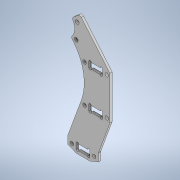
# Autodesk Inventor part: 頭_メインフレーム
Saved by Autodesk Inventor 2020 (Build 240168000, 168)
## iProperties
Created: 2021-09-02
Part Number: 頭_メインフレーム
Material: 一般
Document SubType Name: Modeling
Designer: Masato
Density: 1 g/cm^3
Appearance: 既定
Author: Masato
Autodesk Inventor part; units mm, degrees
ref_plane "YZ Plane" through (0, 0, 0) normal (1, 0, 0) x (0, 1, 0)
ref_plane "XZ Plane" through (0, 0, 0) normal (0, 1, 0) x (-1, 0, 0)
ref_plane "XY Plane" through (0, 0, 0) normal (0, 0, 1) x (1, 0, 0)
sketch "スケッチ1" plane through (0, 0, 0) normal (0, 0, 1) x (1, 0, 0)
  line L0 (0, 0) -> (27, 0) construction
  line L1 (27, 0) -> (27, 5) construction
  line L2 (27, 5) -> (0, 5) construction
  line L3 (0, 5) -> (0, 0) construction
  line L4 (0, 2.5) -> (27, 2.5) construction
  line L5 (13.5, 5) -> (13.5, 0) construction
  circle A0 centre (3.7, 2.5) radius 1.55
  line L6 (7.5, 5) -> (7.5, 0) construction
  circle A1 centre (23.3, 2.5) radius 1.55
  line L7 (19.5, 5) -> (19.5, 0) construction
  line L8 (7.49, 5.01) -> (9.59, 5.01) construction
  line L9 (19.51, 5.01) -> (19.51, -0.01)
  line L10 (19.51, -0.01) -> (17.41, -0.01) construction
  line L11 (7.49, -0.01) -> (7.49, 5.01)
  line L12 (7.49, 5.01) -> (19.51, -0.01) construction
  line L13 (19.51, 5.01) -> (7.49, -0.01) construction
  line L14 (0, 0) -> (7.5, -3)
  line L15 (7.5, -3) -> (19.5, -3)
  line L16 (27, 0) -> (19.5, -3)
  arc A2 (9.59, 5.01) -> (7.49, 5.01) centre (8.54, 5.01) ccw
  arc A3 (7.49, -0.01) -> (9.59, -0.01) centre (8.54, -0.01) ccw
  arc A4 (19.51, 5.01) -> (17.41, 5.01) centre (18.46, 5.01) ccw
  arc A5 (17.41, -0.01) -> (19.51, -0.01) centre (18.46, -0.01) ccw
  line L17 (9.59, 5.01) -> (17.41, 5.01)
  line L18 (9.59, -0.01) -> (7.49, -0.01) construction
  line L19 (17.41, 5.01) -> (19.51, 5.01) construction
  line L20 (17.41, -0.01) -> (9.59, -0.01)
  line L21 (27, 7) -> (0, 7) construction
  line L22 (0, 0) -> (0, 7)
  line L23 (12.1912, 35) -> (37.1912, 35) construction
  line L24 (37.1912, 35) -> (37.1912, 40) construction
  line L25 (37.1912, 40) -> (12.1912, 40) construction
  line L26 (12.1912, 40) -> (12.1912, 35) construction
  line L27 (12.1912, 37.5) -> (37.1912, 37.5) construction
  line L28 (24.6912, 40) -> (24.6912, 35) construction
  circle A6 centre (14.8912, 37.5) radius 1.55
  line L29 (18.6912, 40) -> (18.6912, 35) construction
  line L30 (30.6912, 40) -> (30.6912, 35) construction
  circle A7 centre (34.4912, 37.5) radius 1.55
  line L31 (18.6812, 40.01) -> (20.7812, 40.01) construction
  line L32 (30.7012, 40.01) -> (30.7012, 34.99)
  line L33 (30.7012, 34.99) -> (28.6012, 34.99) construction
  line L34 (18.6812, 34.99) -> (18.6812, 40.01)
  line L35 (18.6812, 40.01) -> (30.7012, 34.99) construction
  line L36 (30.7012, 40.01) -> (18.6812, 34.99) construction
  arc A8 (20.7812, 40.01) -> (18.6812, 40.01) centre (19.7312, 40.01) ccw
  arc A9 (18.6812, 34.99) -> (20.7812, 34.99) centre (19.7312, 34.99) ccw
  arc A10 (30.7012, 40.01) -> (28.6012, 40.01) centre (29.6512, 40.01) ccw
  arc A11 (28.6012, 34.99) -> (30.7012, 34.99) centre (29.6512, 34.99) ccw
  line L37 (20.7812, 40.01) -> (28.6012, 40.01)
  line L38 (20.7812, 34.99) -> (18.6812, 34.99) construction
  line L39 (28.6012, 40.01) -> (30.7012, 40.01) construction
  line L40 (28.6012, 34.99) -> (20.7812, 34.99)
  line L41 (12.1912, 73) -> (12.1912, 68) construction
  circle A12 centre (14.8912, 70.5) radius 1.55
  line L42 (37.1912, 68) -> (37.1912, 73) construction
  line L43 (30.6912, 73) -> (30.6912, 68) construction
  circle A13 centre (34.4912, 70.5) radius 1.55
  line L44 (30.7012, 73.01) -> (30.7012, 67.99)
  line L45 (18.6912, 73) -> (18.6912, 68) construction
  line L46 (12.1912, 68) -> (37.1912, 68) construction
  line L47 (37.1912, 73) -> (12.1912, 73) construction
  line L48 (12.1912, 70.5) -> (37.1912, 70.5) construction
  line L49 (24.6912, 73) -> (24.6912, 68) construction
  line L50 (20.7812, 73.01) -> (28.6012, 73.01)
  line L51 (28.6012, 67.99) -> (20.7812, 67.99)
  line L52 (18.6812, 73.01) -> (30.7012, 67.99) construction
  line L53 (30.7012, 73.01) -> (18.6812, 67.99) construction
  arc A14 (30.7012, 73.01) -> (28.6012, 73.01) centre (29.6512, 73.01) ccw
  line L54 (28.6012, 73.01) -> (30.7012, 73.01) construction
  arc A15 (28.6012, 67.99) -> (30.7012, 67.99) centre (29.6512, 67.99) ccw
  line L55 (30.7012, 67.99) -> (28.6012, 67.99) construction
  line L56 (18.6812, 73.01) -> (20.7812, 73.01) construction
  line L57 (20.7812, 67.99) -> (18.6812, 67.99) construction
  arc A16 (20.7812, 73.01) -> (18.6812, 73.01) centre (19.7312, 73.01) ccw
  arc A17 (18.6812, 67.99) -> (20.7812, 67.99) centre (19.7312, 67.99) ccw
  line L58 (18.6812, 67.99) -> (18.6812, 73.01)
  line L59 (27, 0) -> (27, 6.6473)
  line L60 (37.1912, 35) -> (27.1206, 7.3314)
  line L61 (11.8992, 39.6929) -> (0, 7)
  line L62 (37.1912, 35) -> (37.1912, 73)
  line L63 (9.1035, 103.3621) -> (4.9463, 99.8738)
  arc A18 (3.8121, 84.8933) -> (4.5202, 97.3071) centre (-4.8938, 91.617) ccw
  circle A19 centre (-4.8938, 91.617) radius 14.6063 construction
  line L64 (1.0459, 61.9185) -> (-21.5815, 84.5459) construction
  line L65 (-21.5815, 84.5459) -> (-18.0459, 88.0815) construction
  line L66 (-18.0459, 88.0815) -> (4.5815, 65.4541) construction
  line L67 (4.5815, 65.4541) -> (1.0459, 61.9185) construction
  line L68 (1.0459, 61.9185) -> (-18.0459, 88.0815) construction
  line L69 (-21.5815, 84.5459) -> (4.5815, 65.4541) construction
  line L70 (11.9212, 103.1156) -> (37.1912, 73)
  arc A20 (11.8992, 39.6929) -> (3.8916, 82.3518) centre (-28.1256, 54.2607) ccw
  arc A21 (8.344, 97.7899) -> (6.2953, 101.0057) centre (-4.8938, 91.617) ccw construction
  arc A22 (5.0756, 80.942) -> (7.4988, 83.886) centre (-4.8938, 91.617) ccw construction
  circle A23 centre (8.344, 97.7899) radius 1.65
  circle A24 centre (7.4988, 83.886) radius 1.65
  arc A25 (11.9212, 103.1156) -> (9.1035, 103.3621) centre (10.3891, 101.83) ccw
  arc A26 (4.9463, 99.8738) -> (4.5202, 97.3071) centre (6.2318, 98.3417) ccw
  arc A27 (3.8121, 84.8933) -> (3.8916, 82.3518) centre (5.395, 83.6708) ccw
  arc A28 (27.1206, 7.3314) -> (27, 6.6473) centre (29, 6.6473) ccw
  point P0 (13.5, 2.5)
  point P1 (24.6912, 37.5)
  point P2 (24.6912, 70.5)
  point P3 (10.6356, 104.6477)
  point P4 (3.5327, 98.6877)
  point P5 (-8.5, 75)
  dimension "d0" = 27
  dimension "d1" = 5
  dimension "d2" = 3.1
  dimension "d3" = 12
  dimension "d4" = 19.6
  dimension "d5" = 0.01
  dimension "d6" = 0.01
  dimension "d7" = 3
  dimension "d8" = 12
  dimension "d9" = 1.05
  dimension "d10" = 7
  dimension "d11" = 25
  dimension "d12" = 5
  dimension "d13" = 3.1
  dimension "d14" = 12
  dimension "d15" = 19.6
  dimension "d16" = 0.01
  dimension "d17" = 0.01
  dimension "d20" = 1.05
  dimension "d22" = 25
  dimension "d23" = 5
  dimension "d24" = 3.1
  dimension "d25" = 12
  dimension "d26" = 19.6
  dimension "d27" = 0.01
  dimension "d28" = 0.01
  dimension "d29" = 1.05
  dimension "d30" = 70
  dimension "d31" = 66
  dimension "d32" = 33
  dimension "d37" = 5
  dimension "d38" = 75
  dimension "d39" = 135
  dimension "d40" = 8.5
  dimension "d46" = 11.8
  dimension "d47" = 32
  dimension "d48" = 50
  dimension "d49" = 6.8
  dimension "d50" = 11
  dimension "d51" = 29.2126
  dimension "d54" = 15
  dimension "d55" = 15
  dimension "d56" = 3.3
  dimension "d57" = 3.3
  dimension "d60" = 2
  dimension "d61" = 2
  constraints: 142 end point, 47 point on circle, 40 parallel, 29 centre point, 28 symmetric about line, 26 midpoint, 18 perpendicular, 18 point on line, 14 horizontal, 9 tangent, 4 equal radius, 3 coincident, 1 collinear, 1 line through centre, 1 vertical, 13 other
  measures "d0" distance of L2.end L1.end
  measures "d1" distance of L1.end L0.end
  measures "d2" diameter of A0
  measures "d3" distance of L7.end L6.end
  measures "d4" distance of A1.centre A0.centre
  measures "d5" horizontal distance of L6.start L8.start
  measures "d6" distance from line of L8 L6.start
  measures "d7" vertical distance of L14.end L0.start
  measures "d8" distance of L14.end L15.end
  measures "d9" radius of A2
  measures "d10" distance of L0.start L21.end
  measures "d11" distance of L26.start L24.end
  measures "d12" distance of L24.end L24.start
  measures "d13" diameter of A6
  measures "d14" distance of L30.end L29.end
  measures "d15" distance of A7.centre A6.centre
  measures "d16" horizontal distance of L29.start L35.start
  measures "d17" distance from line of L31 L29.start
  measures "d20" radius of A8
  measures "d22" distance of L47.start L47.end
  measures "d23" distance of L47.start L46.end
  measures "d24" diameter of A12
  measures "d25" distance of L43.end L45.end
  measures "d26" distance of A13.centre A12.centre
  measures "d27" horizontal distance of L45.start L58.end
  measures "d28" distance from line of L56 L45.start
  measures "d29" radius of A16
  measures "d30" angle of L21 L60
  measures "d31" vertical distance of L47.start L21.start
  measures "d32" vertical distance of L21.start L24.end
  measures "d37" distance of L64.end L65.end
  measures "d38" vertical distance of point (-8.5, 75) L0.start
  measures "d39" angle of L64 L3
  measures "d40" horizontal distance of L0.start point (-8.5, 75)
  measures "d46" distance from line of A19.centre L66
  measures "d47" distance of L64.start L64.end
  measures "d48" angle of L0 L70
  measures "d49" distance from line of A18.centre L65
  measures "d50" radius of A18
  measures "d51" diameter of A19
  measures "d56" diameter of A23
  measures "d57" diameter of A24
  measures "d60" radius of A25
  measures "d61" radius of A28
extrude "押し出し1" add sketch "スケッチ1" against normal blind 2
equation "\"d5\" = d6"
equation "\"d12\" = d1"
equation "\"d13\" = d2"
equation "\"d14\" = d3"
equation "\"d15\" = d4"
equation "\"d16\" = d6"
equation "\"d17\" = d6"
equation "\"d22\" = d11"
equation "\"d23\" = d1"
equation "\"d24\" = d2"
equation "\"d25\" = d3"
equation "\"d26\" = d4"
equation "\"d27\" = d6"
equation "\"d28\" = d6"
equation "\"d32\" = 0.5 * d31"
